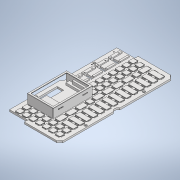
# Autodesk Inventor part: Backboard
Saved by Autodesk Inventor 2021 (Build 250183000, 183)
## iProperties
Created: 2020-06-05
Part Number: Backboard
Material: Generic
Document SubType Name: Modeling
Designer: ameli
Density: 1 g/cm^3
Appearance: Default
Author: ameli
Autodesk Inventor part; units mm, degrees
(part 1 of 4)
ref_plane "YZ Plane" through (0, 0, 0) normal (1, 0, 0) x (0, 1, 0)
ref_plane "XZ Plane" through (0, 0, 0) normal (0, 1, 0) x (-1, 0, 0)
sketch "Sketch1" plane through (0, 0, 0) normal (0, 1, 0) x (-1, 0, 0)
  line L0 (60.5, 128.25) -> (-60.5, 128.25)
  line L1 (-60.5, 128.25) -> (-60.5, -128.25)
  line L2 (-60.5, -128.25) -> (60.5, -128.25)
  line L3 (60.5, -128.25) -> (60.5, 128.25)
  point P0 (0, 0)
  dimension "d0" = 121
  dimension "d1" = 256.5
  dimension "d2" = 60.5
  dimension "d3" = 128.25
  constraints: 8 end point, 2 parallel, 1 horizontal, 1 perpendicular
  measures "d0" distance of L0.start L0.end
  measures "d1" distance of L2.end L0.start
  measures "d2" distance from line of point (0, 0) L3
  measures "d3" distance from line of point (0, 0) L0
extrude "Extrusion1" add sketch "Sketch1" along normal blind 4
sketch "Sketch10" plane through (0, 4, 0) normal (0, 1, 0) x (1, 0, 0)
  line L0 (-49.5, -119.5) -> (-41, -119.5)
  line L1 (-41, -119.5) -> (-41, -118)
  line L2 (-41, -118) -> (-49.5, -118)
  line L3 (-49.5, -118) -> (-49.5, -119.5)
  line L4 (-49.5, -107) -> (-41, -107)
  line L5 (-41, -107) -> (-41, -105.5)
  line L6 (-41, -105.5) -> (-49.5, -105.5)
  line L7 (-49.5, -105.5) -> (-49.5, -107)
  line L8 (-60.5, 128.25) -> (-60.5, -128.25) projected
  line L9 (-60.5, -128.25) -> (60.5, -128.25) projected
  line L10 (-49.5, -104.5) -> (-41, -104.5)
  line L11 (-41, -104.5) -> (-41, -103)
  line L12 (-41, -103) -> (-49.5, -103)
  line L13 (-49.5, -103) -> (-49.5, -104.5)
  line L14 (-49.5, -92) -> (-41, -92)
  line L15 (-41, -92) -> (-41, -90.5)
  line L16 (-41, -90.5) -> (-49.5, -90.5)
  line L17 (-49.5, -90.5) -> (-49.5, -92)
  line L18 (-49.5, -89.5) -> (-41, -89.5)
  line L19 (-41, -89.5) -> (-41, -88)
  line L20 (-41, -88) -> (-49.5, -88)
  line L21 (-49.5, -88) -> (-49.5, -89.5)
  line L22 (-49.5, -77) -> (-41, -77)
  line L23 (-41, -77) -> (-41, -75.5)
  line L24 (-41, -75.5) -> (-49.5, -75.5)
  line L25 (-49.5, -75.5) -> (-49.5, -77)
  line L26 (-49.5, -74.5) -> (-41, -74.5)
  line L27 (-41, -74.5) -> (-41, -73)
  line L28 (-41, -73) -> (-49.5, -73)
  line L29 (-49.5, -73) -> (-49.5, -74.5)
  line L30 (-49.5, -62) -> (-41, -62)
  line L31 (-41, -62) -> (-41, -60.5)
  line L32 (-41, -60.5) -> (-49.5, -60.5)
  line L33 (-49.5, -60.5) -> (-49.5, -62)
  line L34 (-49.5, -59.5) -> (-41, -59.5)
  line L35 (-41, -59.5) -> (-41, -58)
  line L36 (-41, -58) -> (-49.5, -58)
  line L37 (-49.5, -58) -> (-49.5, -59.5)
  line L38 (-49.5, -47) -> (-41, -47)
  line L39 (-41, -47) -> (-41, -45.5)
  line L40 (-41, -45.5) -> (-49.5, -45.5)
  line L41 (-49.5, -45.5) -> (-49.5, -47)
  line L42 (-49.5, -44.5) -> (-41, -44.5)
  line L43 (-41, -44.5) -> (-41, -43)
  line L44 (-41, -43) -> (-49.5, -43)
  line L45 (-49.5, -43) -> (-49.5, -44.5)
  line L46 (-49.5, -32) -> (-41, -32)
  line L47 (-41, -32) -> (-41, -30.5)
  line L48 (-41, -30.5) -> (-49.5, -30.5)
  line L49 (-49.5, -30.5) -> (-49.5, -32)
  line L50 (-49.5, -29.5) -> (-41, -29.5)
  line L51 (-41, -29.5) -> (-41, -28)
  line L52 (-41, -28) -> (-49.5, -28)
  line L53 (-49.5, -28) -> (-49.5, -29.5)
  line L54 (-49.5, -17) -> (-41, -17)
  line L55 (-41, -17) -> (-41, -15.5)
  line L56 (-41, -15.5) -> (-49.5, -15.5)
  line L57 (-49.5, -15.5) -> (-49.5, -17)
  line L58 (-49.5, -14.5) -> (-41, -14.5)
  line L59 (-41, -14.5) -> (-41, -13)
  line L60 (-41, -13) -> (-49.5, -13)
  line L61 (-49.5, -13) -> (-49.5, -14.5)
  line L62 (-49.5, -2) -> (-41, -2)
  line L63 (-41, -2) -> (-41, -0.5)
  line L64 (-41, -0.5) -> (-49.5, -0.5)
  line L65 (-49.5, -0.5) -> (-49.5, -2)
  line L66 (-49.5, 0.5) -> (-41, 0.5)
  line L67 (-41, 0.5) -> (-41, 2)
  line L68 (-41, 2) -> (-49.5, 2)
  line L69 (-49.5, 2) -> (-49.5, 0.5)
  line L70 (-49.5, 13) -> (-41, 13)
  line L71 (-41, 13) -> (-41, 14.5)
  line L72 (-41, 14.5) -> (-49.5, 14.5)
  line L73 (-49.5, 14.5) -> (-49.5, 13)
  line L74 (-49.5, 15.5) -> (-41, 15.5)
  line L75 (-41, 15.5) -> (-41, 17)
  line L76 (-41, 17) -> (-49.5, 17)
  line L77 (-49.5, 17) -> (-49.5, 15.5)
  line L78 (-49.5, 28) -> (-41, 28)
  line L79 (-41, 28) -> (-41, 29.5)
  line L80 (-41, 29.5) -> (-49.5, 29.5)
  line L81 (-49.5, 29.5) -> (-49.5, 28)
  line L82 (-49.5, 30.5) -> (-41, 30.5)
  line L83 (-41, 30.5) -> (-41, 32)
  line L84 (-41, 32) -> (-49.5, 32)
  line L85 (-49.5, 32) -> (-49.5, 30.5)
  line L86 (-49.5, 43) -> (-41, 43)
  line L87 (-41, 43) -> (-41, 44.5)
  line L88 (-41, 44.5) -> (-49.5, 44.5)
  line L89 (-49.5, 44.5) -> (-49.5, 43)
  line L90 (-49.5, 45.5) -> (-41, 45.5)
  line L91 (-41, 45.5) -> (-41, 47)
  line L92 (-41, 47) -> (-49.5, 47)
  line L93 (-49.5, 47) -> (-49.5, 45.5)
  line L94 (-49.5, 58) -> (-41, 58)
  line L95 (-41, 58) -> (-41, 59.5)
  line L96 (-41, 59.5) -> (-49.5, 59.5)
  line L97 (-49.5, 59.5) -> (-49.5, 58)
  line L98 (-49.5, 60.5) -> (-41, 60.5)
  line L99 (-41, 60.5) -> (-41, 62)
  line L100 (-41, 62) -> (-49.5, 62)
  line L101 (-49.5, 62) -> (-49.5, 60.5)
  line L102 (-49.5, 73) -> (-41, 73)
  line L103 (-41, 73) -> (-41, 74.5)
  line L104 (-41, 74.5) -> (-49.5, 74.5)
  line L105 (-49.5, 74.5) -> (-49.5, 73)
  line L106 (-49.5, 75.5) -> (-41, 75.5)
  line L107 (-41, 75.5) -> (-41, 77)
  line L108 (-41, 77) -> (-49.5, 77)
  line L109 (-49.5, 77) -> (-49.5, 75.5)
  line L110 (-49.5, 88) -> (-41, 88)
  line L111 (-41, 88) -> (-41, 89.5)
  line L112 (-41, 89.5) -> (-49.5, 89.5)
  line L113 (-49.5, 89.5) -> (-49.5, 88)
  line L114 (-49.5, 90.5) -> (-41, 90.5)
  line L115 (-41, 90.5) -> (-41, 92)
  line L116 (-41, 92) -> (-49.5, 92)
  line L117 (-49.5, 92) -> (-49.5, 90.5)
  line L118 (-49.5, 103) -> (-41, 103)
  line L119 (-41, 103) -> (-41, 104.5)
  line L120 (-41, 104.5) -> (-49.5, 104.5)
  line L121 (-49.5, 104.5) -> (-49.5, 103)
  line L122 (-49.5, 105.5) -> (-41, 105.5)
  line L123 (-41, 105.5) -> (-41, 107)
  line L124 (-41, 107) -> (-49.5, 107)
  line L125 (-49.5, 107) -> (-49.5, 105.5)
  line L126 (-49.5, 118) -> (-41, 118)
  line L127 (-41, 118) -> (-41, 119.5)
  line L128 (-41, 119.5) -> (-49.5, 119.5)
  line L129 (-49.5, 119.5) -> (-49.5, 118)
  line L130 (-34.5, -119.5) -> (-26, -119.5)
  line L131 (-26, -119.5) -> (-26, -118)
  line L132 (-26, -118) -> (-34.5, -118)
  line L133 (-34.5, -118) -> (-34.5, -119.5)
  line L134 (-34.5, -107) -> (-26, -107)
  line L135 (-26, -107) -> (-26, -105.5)
  line L136 (-26, -105.5) -> (-34.5, -105.5)
  line L137 (-34.5, -105.5) -> (-34.5, -107)
  line L138 (-34.5, -104.5) -> (-26, -104.5)
  line L139 (-26, -104.5) -> (-26, -103)
  line L140 (-26, -103) -> (-34.5, -103)
  line L141 (-34.5, -103) -> (-34.5, -104.5)
  line L142 (-34.5, -92) -> (-26, -92)
  line L143 (-26, -92) -> (-26, -90.5)
  line L144 (-26, -90.5) -> (-34.5, -90.5)
  line L145 (-34.5, -90.5) -> (-34.5, -92)
  line L146 (-34.5, -89.5) -> (-26, -89.5)
  line L147 (-26, -89.5) -> (-26, -88)
  line L148 (-26, -88) -> (-34.5, -88)
  line L149 (-34.5, -88) -> (-34.5, -89.5)
  line L150 (-34.5, -77) -> (-26, -77)
  line L151 (-26, -77) -> (-26, -75.5)
  line L152 (-26, -75.5) -> (-34.5, -75.5)
  line L153 (-34.5, -75.5) -> (-34.5, -77)
  line L154 (-34.5, -74.5) -> (-26, -74.5)
  line L155 (-26, -74.5) -> (-26, -73)
  line L156 (-26, -73) -> (-34.5, -73)
  line L157 (-34.5, -73) -> (-34.5, -74.5)
  line L158 (-34.5, -62) -> (-26, -62)
  line L159 (-26, -62) -> (-26, -60.5)
  line L160 (-26, -60.5) -> (-34.5, -60.5)
  line L161 (-34.5, -60.5) -> (-34.5, -62)
  line L162 (-34.5, -59.5) -> (-26, -59.5)
  line L163 (-26, -59.5) -> (-26, -58)
  line L164 (-26, -58) -> (-34.5, -58)
  line L165 (-34.5, -58) -> (-34.5, -59.5)
  line L166 (-34.5, -47) -> (-26, -47)
  line L167 (-26, -47) -> (-26, -45.5)
  line L168 (-26, -45.5) -> (-34.5, -45.5)
  line L169 (-34.5, -45.5) -> (-34.5, -47)
  line L170 (-34.5, -44.5) -> (-26, -44.5)
  line L171 (-26, -44.5) -> (-26, -43)
  line L172 (-26, -43) -> (-34.5, -43)
  line L173 (-34.5, -43) -> (-34.5, -44.5)
  line L174 (-34.5, -32) -> (-26, -32)
  line L175 (-26, -32) -> (-26, -30.5)
  line L176 (-26, -30.5) -> (-34.5, -30.5)
  line L177 (-34.5, -30.5) -> (-34.5, -32)
  line L178 (-34.5, -29.5) -> (-26, -29.5)
  line L179 (-26, -29.5) -> (-26, -28)
  line L180 (-26, -28) -> (-34.5, -28)
  line L181 (-34.5, -28) -> (-34.5, -29.5)
  line L182 (-34.5, -17) -> (-26, -17)
  line L183 (-26, -17) -> (-26, -15.5)
  line L184 (-26, -15.5) -> (-34.5, -15.5)
  line L185 (-34.5, -15.5) -> (-34.5, -17)
  line L186 (-34.5, -14.5) -> (-26, -14.5)
  line L187 (-26, -14.5) -> (-26, -13)
  line L188 (-26, -13) -> (-34.5, -13)
  line L189 (-34.5, -13) -> (-34.5, -14.5)
  line L190 (-34.5, -2) -> (-26, -2)
  line L191 (-26, -2) -> (-26, -0.5)
  line L192 (-26, -0.5) -> (-34.5, -0.5)
  line L193 (-34.5, -0.5) -> (-34.5, -2)
  line L194 (-34.5, 0.5) -> (-26, 0.5)
  line L195 (-26, 0.5) -> (-26, 2)
  line L196 (-26, 2) -> (-34.5, 2)
  line L197 (-34.5, 2) -> (-34.5, 0.5)
  line L198 (-34.5, 13) -> (-26, 13)
  line L199 (-26, 13) -> (-26, 14.5)
  line L200 (-26, 14.5) -> (-34.5, 14.5)
  line L201 (-34.5, 14.5) -> (-34.5, 13)
  line L202 (-34.5, 15.5) -> (-26, 15.5)
  line L203 (-26, 15.5) -> (-26, 17)
  line L204 (-26, 17) -> (-34.5, 17)
  line L205 (-34.5, 17) -> (-34.5, 15.5)
  line L206 (-34.5, 28) -> (-26, 28)
  line L207 (-26, 28) -> (-26, 29.5)
  line L208 (-26, 29.5) -> (-34.5, 29.5)
  line L209 (-34.5, 29.5) -> (-34.5, 28)
  line L210 (-34.5, 30.5) -> (-26, 30.5)
  line L211 (-26, 30.5) -> (-26, 32)
  line L212 (-26, 32) -> (-34.5, 32)
  line L213 (-34.5, 32) -> (-34.5, 30.5)
  line L214 (-34.5, 43) -> (-26, 43)
  line L215 (-26, 43) -> (-26, 44.5)
  line L216 (-26, 44.5) -> (-34.5, 44.5)
  line L217 (-34.5, 44.5) -> (-34.5, 43)
  line L218 (-34.5, 45.5) -> (-26, 45.5)
  line L219 (-26, 45.5) -> (-26, 47)
  line L220 (-26, 47) -> (-34.5, 47)
  line L221 (-34.5, 47) -> (-34.5, 45.5)
  line L222 (-34.5, 58) -> (-26, 58)
  line L223 (-26, 58) -> (-26, 59.5)
  line L224 (-26, 59.5) -> (-34.5, 59.5)
  line L225 (-34.5, 59.5) -> (-34.5, 58)
  line L226 (-34.5, 60.5) -> (-26, 60.5)
  line L227 (-26, 60.5) -> (-26, 62)
  line L228 (-26, 62) -> (-34.5, 62)
  line L229 (-34.5, 62) -> (-34.5, 60.5)
  line L230 (-34.5, 73) -> (-26, 73)
  line L231 (-26, 73) -> (-26, 74.5)
  line L232 (-26, 74.5) -> (-34.5, 74.5)
  line L233 (-34.5, 74.5) -> (-34.5, 73)
  line L234 (-34.5, 75.5) -> (-26, 75.5)
  line L235 (-26, 75.5) -> (-26, 77)
  line L236 (-26, 77) -> (-34.5, 77)
  line L237 (-34.5, 77) -> (-34.5, 75.5)
  line L238 (-34.5, 88) -> (-26, 88)
  line L239 (-26, 88) -> (-26, 89.5)
  line L240 (-26, 89.5) -> (-34.5, 89.5)
  line L241 (-34.5, 89.5) -> (-34.5, 88)
  line L242 (-34.5, 90.5) -> (-26, 90.5)
  line L243 (-26, 90.5) -> (-26, 92)
  line L244 (-26, 92) -> (-34.5, 92)
  line L245 (-34.5, 92) -> (-34.5, 90.5)
  line L246 (-34.5, 103) -> (-26, 103)
  line L247 (-26, 103) -> (-26, 104.5)
  line L248 (-26, 104.5) -> (-34.5, 104.5)
  line L249 (-34.5, 104.5) -> (-34.5, 103)
  line L250 (-34.5, 105.5) -> (-26, 105.5)
  line L251 (-26, 105.5) -> (-26, 107)
  line L252 (-26, 107) -> (-34.5, 107)
  line L253 (-34.5, 107) -> (-34.5, 105.5)
  line L254 (-34.5, 118) -> (-26, 118)
  line L255 (-26, 118) -> (-26, 119.5)
  line L256 (-26, 119.5) -> (-34.5, 119.5)
  line L257 (-34.5, 119.5) -> (-34.5, 118)
  line L258 (-19.5, -119.5) -> (-11, -119.5)
  line L259 (-11, -119.5) -> (-11, -118)
  line L260 (-11, -118) -> (-19.5, -118)
  line L261 (-19.5, -118) -> (-19.5, -119.5)
  line L262 (-19.5, -107) -> (-11, -107)
  line L263 (-11, -107) -> (-11, -105.5)
  line L264 (-11, -105.5) -> (-19.5, -105.5)
  line L265 (-19.5, -105.5) -> (-19.5, -107)
  line L266 (-19.5, -104.5) -> (-11, -104.5)
  line L267 (-11, -104.5) -> (-11, -103)
  line L268 (-11, -103) -> (-19.5, -103)
  line L269 (-19.5, -103) -> (-19.5, -104.5)
  line L270 (-19.5, -92) -> (-11, -92)
  line L271 (-11, -92) -> (-11, -90.5)
  line L272 (-11, -90.5) -> (-19.5, -90.5)
  line L273 (-19.5, -90.5) -> (-19.5, -92)
  line L274 (-19.5, -89.5) -> (-11, -89.5)
  line L275 (-11, -89.5) -> (-11, -88)
  line L276 (-11, -88) -> (-19.5, -88)
  line L277 (-19.5, -88) -> (-19.5, -89.5)
  line L278 (-19.5, -77) -> (-11, -77)
  line L279 (-11, -77) -> (-11, -75.5)
  line L280 (-11, -75.5) -> (-19.5, -75.5)
  line L281 (-19.5, -75.5) -> (-19.5, -77)
  line L282 (-19.5, -74.5) -> (-11, -74.5)
  line L283 (-11, -74.5) -> (-11, -73)
  line L284 (-11, -73) -> (-19.5, -73)
  line L285 (-19.5, -73) -> (-19.5, -74.5)
  line L286 (-19.5, -62) -> (-11, -62)
  line L287 (-11, -62) -> (-11, -60.5)
  line L288 (-11, -60.5) -> (-19.5, -60.5)
  line L289 (-19.5, -60.5) -> (-19.5, -62)
  line L290 (-19.5, -59.5) -> (-11, -59.5)
  line L291 (-11, -59.5) -> (-11, -58)
  line L292 (-11, -58) -> (-19.5, -58)
  line L293 (-19.5, -58) -> (-19.5, -59.5)
  line L294 (-19.5, -47) -> (-11, -47)
  line L295 (-11, -47) -> (-11, -45.5)
  line L296 (-11, -45.5) -> (-19.5, -45.5)
  line L297 (-19.5, -45.5) -> (-19.5, -47)
  line L298 (-19.5, -44.5) -> (-11, -44.5)
  line L299 (-11, -44.5) -> (-11, -43)
  line L300 (-11, -43) -> (-19.5, -43)
  line L301 (-19.5, -43) -> (-19.5, -44.5)
  line L302 (-19.5, -32) -> (-11, -32)
  line L303 (-11, -32) -> (-11, -30.5)
  line L304 (-11, -30.5) -> (-19.5, -30.5)
  line L305 (-19.5, -30.5) -> (-19.5, -32)
  line L306 (-19.5, -29.5) -> (-11, -29.5)
  line L307 (-11, -29.5) -> (-11, -28)
  line L308 (-11, -28) -> (-19.5, -28)
  line L309 (-19.5, -28) -> (-19.5, -29.5)
  line L310 (-19.5, -17) -> (-11, -17)
  line L311 (-11, -17) -> (-11, -15.5)
  line L312 (-11, -15.5) -> (-19.5, -15.5)
  line L313 (-19.5, -15.5) -> (-19.5, -17)
  line L314 (-19.5, -14.5) -> (-11, -14.5)
  line L315 (-11, -14.5) -> (-11, -13)
  line L316 (-11, -13) -> (-19.5, -13)
  line L317 (-19.5, -13) -> (-19.5, -14.5)
  line L318 (-19.5, -2) -> (-11, -2)
  line L319 (-11, -2) -> (-11, -0.5)
  line L320 (-11, -0.5) -> (-19.5, -0.5)
  line L321 (-19.5, -0.5) -> (-19.5, -2)
  line L322 (-19.5, 0.5) -> (-11, 0.5)
  line L323 (-11, 0.5) -> (-11, 2)
  line L324 (-11, 2) -> (-19.5, 2)
  line L325 (-19.5, 2) -> (-19.5, 0.5)
  line L326 (-19.5, 13) -> (-11, 13)
  line L327 (-11, 13) -> (-11, 14.5)
  line L328 (-11, 14.5) -> (-19.5, 14.5)
  line L329 (-19.5, 14.5) -> (-19.5, 13)
  line L330 (-19.5, 15.5) -> (-11, 15.5)
  line L331 (-11, 15.5) -> (-11, 17)
  line L332 (-11, 17) -> (-19.5, 17)
  line L333 (-19.5, 17) -> (-19.5, 15.5)
  line L334 (-19.5, 28) -> (-11, 28)
  line L335 (-11, 28) -> (-11, 29.5)
  line L336 (-11, 29.5) -> (-19.5, 29.5)
  line L337 (-19.5, 29.5) -> (-19.5, 28)
  line L338 (-19.5, 30.5) -> (-11, 30.5)
  line L339 (-11, 30.5) -> (-11, 32)
  line L340 (-11, 32) -> (-19.5, 32)
  line L341 (-19.5, 32) -> (-19.5, 30.5)
  line L342 (-19.5, 43) -> (-11, 43)
  line L343 (-11, 43) -> (-11, 44.5)
  line L344 (-11, 44.5) -> (-19.5, 44.5)
  line L345 (-19.5, 44.5) -> (-19.5, 43)
  line L346 (-19.5, 45.5) -> (-11, 45.5)
  line L347 (-11, 45.5) -> (-11, 47)
  line L348 (-11, 47) -> (-19.5, 47)
  line L349 (-19.5, 47) -> (-19.5, 45.5)
  line L350 (-19.5, 58) -> (-11, 58)
  line L351 (-11, 58) -> (-11, 59.5)
  line L352 (-11, 59.5) -> (-19.5, 59.5)
  line L353 (-19.5, 59.5) -> (-19.5, 58)
  line L354 (-19.5, 60.5) -> (-11, 60.5)
  line L355 (-11, 60.5) -> (-11, 62)
  line L356 (-11, 62) -> (-19.5, 62)
  line L357 (-19.5, 62) -> (-19.5, 60.5)
  line L358 (-19.5, 73) -> (-11, 73)
  line L359 (-11, 73) -> (-11, 74.5)
  line L360 (-11, 74.5) -> (-19.5, 74.5)
  line L361 (-19.5, 74.5) -> (-19.5, 73)
  line L362 (-19.5, 75.5) -> (-11, 75.5)
  line L363 (-11, 75.5) -> (-11, 77)
  line L364 (-11, 77) -> (-19.5, 77)
  line L365 (-19.5, 77) -> (-19.5, 75.5)
  line L366 (-19.5, 88) -> (-11, 88)
  line L367 (-11, 88) -> (-11, 89.5)
  line L368 (-11, 89.5) -> (-19.5, 89.5)
  line L369 (-19.5, 89.5) -> (-19.5, 88)
  line L370 (-19.5, 90.5) -> (-11, 90.5)
  line L371 (-11, 90.5) -> (-11, 92)
  line L372 (-11, 92) -> (-19.5, 92)
  line L373 (-19.5, 92) -> (-19.5, 90.5)
  line L374 (-19.5, 103) -> (-11, 103)
  line L375 (-11, 103) -> (-11, 104.5)
  line L376 (-11, 104.5) -> (-19.5, 104.5)
  line L377 (-19.5, 104.5) -> (-19.5, 103)
  line L378 (-19.5, 105.5) -> (-11, 105.5)
  line L379 (-11, 105.5) -> (-11, 107)
  line L380 (-11, 107) -> (-19.5, 107)
  line L381 (-19.5, 107) -> (-19.5, 105.5)
  line L382 (-19.5, 118) -> (-11, 118)
  line L383 (-11, 118) -> (-11, 119.5)
  line L384 (-11, 119.5) -> (-19.5, 119.5)
  line L385 (-19.5, 119.5) -> (-19.5, 118)
  line L386 (-4.5, -119.5) -> (4, -119.5)
  line L387 (4, -119.5) -> (4, -118)
  line L388 (4, -118) -> (-4.5, -118)
  line L389 (-4.5, -118) -> (-4.5, -119.5)
  line L390 (-4.5, -107) -> (4, -107)
  line L391 (4, -107) -> (4, -105.5)
  line L392 (4, -105.5) -> (-4.5, -105.5)
  line L393 (-4.5, -105.5) -> (-4.5, -107)
  line L394 (-4.5, -104.5) -> (4, -104.5)
  line L395 (4, -104.5) -> (4, -103)
  line L396 (4, -103) -> (-4.5, -103)
  line L397 (-4.5, -103) -> (-4.5, -104.5)
  line L398 (-4.5, -92) -> (4, -92)
  line L399 (4, -92) -> (4, -90.5)
  line L400 (4, -90.5) -> (-4.5, -90.5)
  line L401 (-4.5, -90.5) -> (-4.5, -92)
  line L402 (-4.5, -89.5) -> (4, -89.5)
  line L403 (4, -89.5) -> (4, -88)
  line L404 (4, -88) -> (-4.5, -88)
  line L405 (-4.5, -88) -> (-4.5, -89.5)
  line L406 (-4.5, -77) -> (4, -77)
  line L407 (4, -77) -> (4, -75.5)
  line L408 (4, -75.5) -> (-4.5, -75.5)
  line L409 (-4.5, -75.5) -> (-4.5, -77)
  line L410 (-4.5, -74.5) -> (4, -74.5)
  line L411 (4, -74.5) -> (4, -73)
  line L412 (4, -73) -> (-4.5, -73)
  line L413 (-4.5, -73) -> (-4.5, -74.5)
  line L414 (-4.5, -62) -> (4, -62)
  line L415 (4, -62) -> (4, -60.5)
  line L416 (4, -60.5) -> (-4.5, -60.5)
  line L417 (-4.5, -60.5) -> (-4.5, -62)
  line L418 (-4.5, -59.5) -> (4, -59.5)
  line L419 (4, -59.5) -> (4, -58)
  line L420 (4, -58) -> (-4.5, -58)
  line L421 (-4.5, -58) -> (-4.5, -59.5)
  line L422 (-4.5, -47) -> (4, -47)
  line L423 (4, -47) -> (4, -45.5)
  line L424 (4, -45.5) -> (-4.5, -45.5)
  line L425 (-4.5, -45.5) -> (-4.5, -47)
  line L426 (-4.5, -44.5) -> (4, -44.5)
  line L427 (4, -44.5) -> (4, -43)
  line L428 (4, -43) -> (-4.5, -43)
  line L429 (-4.5, -43) -> (-4.5, -44.5)
  line L430 (-4.5, -32) -> (4, -32)
  line L431 (4, -32) -> (4, -30.5)
  line L432 (4, -30.5) -> (-4.5, -30.5)
  line L433 (-4.5, -30.5) -> (-4.5, -32)
  line L434 (-4.5, -29.5) -> (4, -29.5)
  line L435 (4, -29.5) -> (4, -28)
  line L436 (4, -28) -> (-4.5, -28)
  line L437 (-4.5, -28) -> (-4.5, -29.5)
  line L438 (-4.5, -17) -> (4, -17)
  line L439 (4, -17) -> (4, -15.5)
  line L440 (4, -15.5) -> (-4.5, -15.5)
  line L441 (-4.5, -15.5) -> (-4.5, -17)
  line L442 (-4.5, -14.5) -> (4, -14.5)
  line L443 (4, -14.5) -> (4, -13)
  line L444 (4, -13) -> (-4.5, -13)
  line L445 (-4.5, -13) -> (-4.5, -14.5)
  line L446 (-4.5, -2) -> (4, -2)
  line L447 (4, -2) -> (4, -0.5)
  line L448 (4, -0.5) -> (-4.5, -0.5)
  line L449 (-4.5, -0.5) -> (-4.5, -2)
  line L450 (-4.5, 0.5) -> (4, 0.5)
  line L451 (4, 0.5) -> (4, 2)
  line L452 (4, 2) -> (-4.5, 2)
  line L453 (-4.5, 2) -> (-4.5, 0.5)
  line L454 (-4.5, 13) -> (4, 13)
  line L455 (4, 13) -> (4, 14.5)
  line L456 (4, 14.5) -> (-4.5, 14.5)
  line L457 (-4.5, 14.5) -> (-4.5, 13)
  line L458 (-4.5, 15.5) -> (4, 15.5)
  line L459 (4, 15.5) -> (4, 17)
  line L460 (4, 17) -> (-4.5, 17)
  line L461 (-4.5, 17) -> (-4.5, 15.5)
  line L462 (-4.5, 28) -> (4, 28)
  line L463 (4, 28) -> (4, 29.5)
  line L464 (4, 29.5) -> (-4.5, 29.5)
  line L465 (-4.5, 29.5) -> (-4.5, 28)
  line L466 (-4.5, 30.5) -> (4, 30.5)
  line L467 (4, 30.5) -> (4, 32)
  line L468 (4, 32) -> (-4.5, 32)
  line L469 (-4.5, 32) -> (-4.5, 30.5)
  line L470 (-4.5, 43) -> (4, 43)
  line L471 (4, 43) -> (4, 44.5)
  line L472 (4, 44.5) -> (-4.5, 44.5)
  line L473 (-4.5, 44.5) -> (-4.5, 43)
  line L474 (-4.5, 45.5) -> (4, 45.5)
  line L475 (4, 45.5) -> (4, 47)
  line L476 (4, 47) -> (-4.5, 47)
  line L477 (-4.5, 47) -> (-4.5, 45.5)
  line L478 (-4.5, 58) -> (4, 58)
  line L479 (4, 58) -> (4, 59.5)
  line L480 (4, 59.5) -> (-4.5, 59.5)
  line L481 (-4.5, 59.5) -> (-4.5, 58)
  line L482 (-4.5, 60.5) -> (4, 60.5)
  line L483 (4, 60.5) -> (4, 62)
  line L484 (4, 62) -> (-4.5, 62)
  line L485 (-4.5, 62) -> (-4.5, 60.5)
  line L486 (-4.5, 73) -> (4, 73)
  line L487 (4, 73) -> (4, 74.5)
  line L488 (4, 74.5) -> (-4.5, 74.5)
  line L489 (-4.5, 74.5) -> (-4.5, 73)
  line L490 (-4.5, 75.5) -> (4, 75.5)
  line L491 (4, 75.5) -> (4, 77)
  line L492 (4, 77) -> (-4.5, 77)
  line L493 (-4.5, 77) -> (-4.5, 75.5)
  line L494 (-4.5, 88) -> (4, 88)
  line L495 (4, 88) -> (4, 89.5)
  line L496 (4, 89.5) -> (-4.5, 89.5)
  line L497 (-4.5, 89.5) -> (-4.5, 88)
  line L498 (-4.5, 90.5) -> (4, 90.5)
  line L499 (4, 90.5) -> (4, 92)
  line L500 (4, 92) -> (-4.5, 92)
  line L501 (-4.5, 92) -> (-4.5, 90.5)
  line L502 (-4.5, 103) -> (4, 103)
  line L503 (4, 103) -> (4, 104.5)
  line L504 (4, 104.5) -> (-4.5, 104.5)
  line L505 (-4.5, 104.5) -> (-4.5, 103)
  line L506 (-4.5, 105.5) -> (4, 105.5)
  line L507 (4, 105.5) -> (4, 107)
  line L508 (4, 107) -> (-4.5, 107)
  line L509 (-4.5, 107) -> (-4.5, 105.5)
  line L510 (-4.5, 118) -> (4, 118)
  line L511 (4, 118) -> (4, 119.5)
  line L512 (4, 119.5) -> (-4.5, 119.5)
  line L513 (-4.5, 119.5) -> (-4.5, 118)
  line L514 (10.5, -119.5) -> (19, -119.5)
  line L515 (19, -119.5) -> (19, -118)
  line L516 (19, -118) -> (10.5, -118)
  line L517 (10.5, -118) -> (10.5, -119.5)
  line L518 (10.5, -107) -> (19, -107)
  line L519 (19, -107) -> (19, -105.5)
  line L520 (19, -105.5) -> (10.5, -105.5)
  line L521 (10.5, -105.5) -> (10.5, -107)
  line L522 (10.5, -104.5) -> (19, -104.5)
  line L523 (19, -104.5) -> (19, -103)
  line L524 (19, -103) -> (10.5, -103)
  line L525 (10.5, -103) -> (10.5, -104.5)
  line L526 (10.5, -92) -> (19, -92)
  line L527 (19, -92) -> (19, -90.5)
  line L528 (19, -90.5) -> (10.5, -90.5)
  line L529 (10.5, -90.5) -> (10.5, -92)
  line L530 (10.5, -89.5) -> (19, -89.5)
  line L531 (19, -89.5) -> (19, -88)
  line L532 (19, -88) -> (10.5, -88)
  line L533 (10.5, -88) -> (10.5, -89.5)
  line L534 (10.5, -77) -> (19, -77)
  line L535 (19, -77) -> (19, -75.5)
  line L536 (19, -75.5) -> (10.5, -75.5)
  line L537 (10.5, -75.5) -> (10.5, -77)
  line L538 (10.5, -74.5) -> (19, -74.5)
  line L539 (19, -74.5) -> (19, -73)
  line L540 (19, -73) -> (10.5, -73)
  line L541 (10.5, -73) -> (10.5, -74.5)
  line L542 (10.5, -62) -> (19, -62)
  line L543 (19, -62) -> (19, -60.5)
  line L544 (19, -60.5) -> (10.5, -60.5)
  line L545 (10.5, -60.5) -> (10.5, -62)
  line L546 (10.5, -59.5) -> (19, -59.5)
  line L547 (19, -59.5) -> (19, -58)
  line L548 (19, -58) -> (10.5, -58)
  line L549 (10.5, -58) -> (10.5, -59.5)
  line L550 (10.5, -47) -> (19, -47)
  line L551 (19, -47) -> (19, -45.5)
  line L552 (19, -45.5) -> (10.5, -45.5)
  line L553 (10.5, -45.5) -> (10.5, -47)
  line L554 (10.5, -44.5) -> (19, -44.5)
  line L555 (19, -44.5) -> (19, -43)
  line L556 (19, -43) -> (10.5, -43)
  line L557 (10.5, -43) -> (10.5, -44.5)
  line L558 (10.5, -32) -> (19, -32)
  line L559 (19, -32) -> (19, -30.5)
  line L560 (19, -30.5) -> (10.5, -30.5)
  line L561 (10.5, -30.5) -> (10.5, -32)
  line L562 (10.5, -29.5) -> (19, -29.5)
  line L563 (19, -29.5) -> (19, -28)
  line L564 (19, -28) -> (10.5, -28)
  line L565 (10.5, -28) -> (10.5, -29.5)
  line L566 (10.5, -17) -> (19, -17)
  line L567 (19, -17) -> (19, -15.5)
  line L568 (19, -15.5) -> (10.5, -15.5)
  line L569 (10.5, -15.5) -> (10.5, -17)
  line L570 (10.5, -14.5) -> (19, -14.5)
  line L571 (19, -14.5) -> (19, -13)
  line L572 (19, -13) -> (10.5, -13)
  line L573 (10.5, -13) -> (10.5, -14.5)
  line L574 (10.5, -2) -> (19, -2)
  line L575 (19, -2) -> (19, -0.5)
  line L576 (19, -0.5) -> (10.5, -0.5)
  line L577 (10.5, -0.5) -> (10.5, -2)
  line L578 (10.5, 0.5) -> (19, 0.5)
  line L579 (19, 0.5) -> (19, 2)
  line L580 (19, 2) -> (10.5, 2)
  line L581 (10.5, 2) -> (10.5, 0.5)
  line L582 (10.5, 13) -> (19, 13)
  line L583 (19, 13) -> (19, 14.5)
  line L584 (19, 14.5) -> (10.5, 14.5)
  line L585 (10.5, 14.5) -> (10.5, 13)
  line L586 (10.5, 15.5) -> (19, 15.5)
  line L587 (19, 15.5) -> (19, 17)
  line L588 (19, 17) -> (10.5, 17)
  line L589 (10.5, 17) -> (10.5, 15.5)
  line L590 (10.5, 28) -> (19, 28)
  line L591 (19, 28) -> (19, 29.5)
  line L592 (19, 29.5) -> (10.5, 29.5)
  line L593 (10.5, 29.5) -> (10.5, 28)
  line L594 (10.5, 30.5) -> (19, 30.5)
  line L595 (19, 30.5) -> (19, 32)
  line L596 (19, 32) -> (10.5, 32)
  line L597 (10.5, 32) -> (10.5, 30.5)
  line L598 (10.5, 43) -> (19, 43)
  line L599 (19, 43) -> (19, 44.5)
  line L600 (19, 44.5) -> (10.5, 44.5)
  line L601 (10.5, 44.5) -> (10.5, 43)
  line L602 (10.5, 45.5) -> (19, 45.5)
  line L603 (19, 45.5) -> (19, 47)
  line L604 (19, 47) -> (10.5, 47)
  line L605 (10.5, 47) -> (10.5, 45.5)
  line L606 (10.5, 58) -> (19, 58)
  line L607 (19, 58) -> (19, 59.5)
  line L608 (19, 59.5) -> (10.5, 59.5)
  line L609 (10.5, 59.5) -> (10.5, 58)
  line L610 (10.5, 60.5) -> (19, 60.5)
  line L611 (19, 60.5) -> (19, 62)
  line L612 (19, 62) -> (10.5, 62)
  line L613 (10.5, 62) -> (10.5, 60.5)
  line L614 (10.5, 73) -> (19, 73)
  line L615 (19, 73) -> (19, 74.5)
  line L616 (19, 74.5) -> (10.5, 74.5)
  line L617 (10.5, 74.5) -> (10.5, 73)
  line L618 (10.5, 75.5) -> (19, 75.5)
  line L619 (19, 75.5) -> (19, 77)
  line L620 (19, 77) -> (10.5, 77)
  line L621 (10.5, 77) -> (10.5, 75.5)
  line L622 (10.5, 88) -> (19, 88)
  line L623 (19, 88) -> (19, 89.5)
  line L624 (19, 89.5) -> (10.5, 89.5)
  line L625 (10.5, 89.5) -> (10.5, 88)
  line L626 (10.5, 90.5) -> (19, 90.5)
  line L627 (19, 90.5) -> (19, 92)
  line L628 (19, 92) -> (10.5, 92)
  line L629 (10.5, 92) -> (10.5, 90.5)
  line L630 (10.5, 103) -> (19, 103)
  line L631 (19, 103) -> (19, 104.5)
  line L632 (19, 104.5) -> (10.5, 104.5)
  line L633 (10.5, 104.5) -> (10.5, 103)
  line L634 (10.5, 105.5) -> (19, 105.5)
  line L635 (19, 105.5) -> (19, 107)
  line L636 (19, 107) -> (10.5, 107)
  line L637 (10.5, 107) -> (10.5, 105.5)
  line L638 (10.5, 118) -> (19, 118)
  line L639 (19, 118) -> (19, 119.5)
  line L640 (19, 119.5) -> (10.5, 119.5)
  line L641 (10.5, 119.5) -> (10.5, 118)
  line L642 (25.5, -119.5) -> (34, -119.5)
  line L643 (34, -119.5) -> (34, -118)
  line L644 (34, -118) -> (25.5, -118)
  line L645 (25.5, -118) -> (25.5, -119.5)
  line L646 (25.5, -107) -> (34, -107)
  line L647 (34, -107) -> (34, -105.5)
  line L648 (34, -105.5) -> (25.5, -105.5)
  line L649 (25.5, -105.5) -> (25.5, -107)
  line L650 (25.5, -104.5) -> (34, -104.5)
  line L651 (34, -104.5) -> (34, -103)
  line L652 (34, -103) -> (25.5, -103)
  line L653 (25.5, -103) -> (25.5, -104.5)
  line L654 (25.5, -92) -> (34, -92)
  line L655 (34, -92) -> (34, -90.5)
  line L656 (34, -90.5) -> (25.5, -90.5)
  line L657 (25.5, -90.5) -> (25.5, -92)
  line L658 (25.5, -89.5) -> (34, -89.5)
  line L659 (34, -89.5) -> (34, -88)
  line L660 (34, -88) -> (25.5, -88)
  line L661 (25.5, -88) -> (25.5, -89.5)
  line L662 (25.5, -77) -> (34, -77)
  line L663 (34, -77) -> (34, -75.5)
  line L664 (34, -75.5) -> (25.5, -75.5)
  line L665 (25.5, -75.5) -> (25.5, -77)
  line L666 (25.5, -74.5) -> (34, -74.5)
  line L667 (34, -74.5) -> (34, -73)
  line L668 (34, -73) -> (25.5, -73)
  line L669 (25.5, -73) -> (25.5, -74.5)
  line L670 (25.5, -62) -> (34, -62)
  line L671 (34, -62) -> (34, -60.5)
  line L672 (34, -60.5) -> (25.5, -60.5)
  line L673 (25.5, -60.5) -> (25.5, -62)
  line L674 (25.5, -59.5) -> (34, -59.5)
  line L675 (34, -59.5) -> (34, -58)
  line L676 (34, -58) -> (25.5, -58)
  line L677 (25.5, -58) -> (25.5, -59.5)
  line L678 (25.5, -47) -> (34, -47)
  line L679 (34, -47) -> (34, -45.5)
  line L680 (34, -45.5) -> (25.5, -45.5)
  line L681 (25.5, -45.5) -> (25.5, -47)
  line L682 (25.5, -44.5) -> (34, -44.5)
  line L683 (34, -44.5) -> (34, -43)
  line L684 (34, -43) -> (25.5, -43)
  line L685 (25.5, -43) -> (25.5, -44.5)
  line L686 (25.5, -32) -> (34, -32)
  line L687 (34, -32) -> (34, -30.5)
  line L688 (34, -30.5) -> (25.5, -30.5)
  line L689 (25.5, -30.5) -> (25.5, -32)
  line L690 (25.5, -29.5) -> (34, -29.5)
  line L691 (34, -29.5) -> (34, -28)
  line L692 (34, -28) -> (25.5, -28)
  line L693 (25.5, -28) -> (25.5, -29.5)
  line L694 (25.5, -17) -> (34, -17)
  line L695 (34, -17) -> (34, -15.5)
  line L696 (34, -15.5) -> (25.5, -15.5)
  line L697 (25.5, -15.5) -> (25.5, -17)
  line L698 (25.5, -14.5) -> (34, -14.5)
  line L699 (34, -14.5) -> (34, -13)
  line L700 (34, -13) -> (25.5, -13)
  line L701 (25.5, -13) -> (25.5, -14.5)
  line L702 (25.5, -2) -> (34, -2)
  line L703 (34, -2) -> (34, -0.5)
  line L704 (34, -0.5) -> (25.5, -0.5)
  line L705 (25.5, -0.5) -> (25.5, -2)
  line L706 (25.5, 0.5) -> (34, 0.5)
  line L707 (34, 0.5) -> (34, 2)
  line L708 (34, 2) -> (25.5, 2)
  line L709 (25.5, 2) -> (25.5, 0.5)
  line L710 (25.5, 13) -> (34, 13)
  line L711 (34, 13) -> (34, 14.5)
  line L712 (34, 14.5) -> (25.5, 14.5)
  line L713 (25.5, 14.5) -> (25.5, 13)
  line L714 (25.5, 15.5) -> (34, 15.5)
  line L715 (34, 15.5) -> (34, 17)
  line L716 (34, 17) -> (25.5, 17)
  line L717 (25.5, 17) -> (25.5, 15.5)
  line L718 (25.5, 28) -> (34, 28)
  line L719 (34, 28) -> (34, 29.5)
  line L720 (34, 29.5) -> (25.5, 29.5)
  line L721 (25.5, 29.5) -> (25.5, 28)
  line L722 (25.5, 30.5) -> (34, 30.5)
  line L723 (34, 30.5) -> (34, 32)
  line L724 (34, 32) -> (25.5, 32)
  line L725 (25.5, 32) -> (25.5, 30.5)
  line L726 (25.5, 43) -> (34, 43)
  line L727 (34, 43) -> (34, 44.5)
  line L728 (34, 44.5) -> (25.5, 44.5)
  line L729 (25.5, 44.5) -> (25.5, 43)
  line L730 (25.5, 45.5) -> (34, 45.5)
  line L731 (34, 45.5) -> (34, 47)
  line L732 (34, 47) -> (25.5, 47)
  line L733 (25.5, 47) -> (25.5, 45.5)
  line L734 (25.5, 58) -> (34, 58)
  line L735 (34, 58) -> (34, 59.5)
  line L736 (34, 59.5) -> (25.5, 59.5)
  line L737 (25.5, 59.5) -> (25.5, 58)
  line L738 (25.5, 60.5) -> (34, 60.5)
  line L739 (34, 60.5) -> (34, 62)
  line L740 (34, 62) -> (25.5, 62)
  line L741 (25.5, 62) -> (25.5, 60.5)
  line L742 (25.5, 73) -> (34, 73)
  line L743 (34, 73) -> (34, 74.5)
  line L744 (34, 74.5) -> (25.5, 74.5)
  line L745 (25.5, 74.5) -> (25.5, 73)
  line L746 (25.5, 75.5) -> (34, 75.5)
  line L747 (34, 75.5) -> (34, 77)
  line L748 (34, 77) -> (25.5, 77)
  line L749 (25.5, 77) -> (25.5, 75.5)
  line L750 (25.5, 88) -> (34, 88)
  line L751 (34, 88) -> (34, 89.5)
  line L752 (34, 89.5) -> (25.5, 89.5)
  line L753 (25.5, 89.5) -> (25.5, 88)
  line L754 (25.5, 90.5) -> (34, 90.5)
  line L755 (34, 90.5) -> (34, 92)
  line L756 (34, 92) -> (25.5, 92)
  line L757 (25.5, 92) -> (25.5, 90.5)
  line L758 (25.5, 103) -> (34, 103)
  line L759 (34, 103) -> (34, 104.5)
  line L760 (34, 104.5) -> (25.5, 104.5)
  line L761 (25.5, 104.5) -> (25.5, 103)
  line L762 (25.5, 105.5) -> (34, 105.5)
  line L763 (34, 105.5) -> (34, 107)
  line L764 (34, 107) -> (25.5, 107)
  line L765 (25.5, 107) -> (25.5, 105.5)
  line L766 (25.5, 118) -> (34, 118)
  line L767 (34, 118) -> (34, 119.5)
  line L768 (34, 119.5) -> (25.5, 119.5)
  line L769 (25.5, 119.5) -> (25.5, 118)
  line L770 (40.5, -119.5) -> (49, -119.5)
  line L771 (49, -119.5) -> (49, -118)
  line L772 (49, -118) -> (40.5, -118)
  line L773 (40.5, -118) -> (40.5, -119.5)
  line L774 (40.5, -107) -> (49, -107)
  line L775 (49, -107) -> (49, -105.5)
  line L776 (49, -105.5) -> (40.5, -105.5)
  line L777 (40.5, -105.5) -> (40.5, -107)
  line L778 (40.5, -104.5) -> (49, -104.5)
  line L779 (49, -104.5) -> (49, -103)
  line L780 (49, -103) -> (40.5, -103)
  line L781 (40.5, -103) -> (40.5, -104.5)
  line L782 (40.5, -92) -> (49, -92)
  line L783 (49, -92) -> (49, -90.5)
  line L784 (49, -90.5) -> (40.5, -90.5)
  line L785 (40.5, -90.5) -> (40.5, -92)
  line L786 (40.5, -89.5) -> (49, -89.5)
  line L787 (49, -89.5) -> (49, -88)
  line L788 (49, -88) -> (40.5, -88)
  line L789 (40.5, -88) -> (40.5, -89.5)
  line L790 (40.5, -77) -> (49, -77)
  line L791 (49, -77) -> (49, -75.5)
  line L792 (49, -75.5) -> (40.5, -75.5)
  line L793 (40.5, -75.5) -> (40.5, -77)
  line L794 (40.5, -74.5) -> (49, -74.5)
  line L795 (49, -74.5) -> (49, -73)
  line L796 (49, -73) -> (40.5, -73)
  line L797 (40.5, -73) -> (40.5, -74.5)
  line L798 (40.5, -62) -> (49, -62)
  line L799 (49, -62) -> (49, -60.5)
  line L800 (49, -60.5) -> (40.5, -60.5)
  line L801 (40.5, -60.5) -> (40.5, -62)
  line L802 (40.5, -59.5) -> (49, -59.5)
  line L803 (49, -59.5) -> (49, -58)
  line L804 (49, -58) -> (40.5, -58)
  line L805 (40.5, -58) -> (40.5, -59.5)
  line L806 (40.5, -47) -> (49, -47)
  line L807 (49, -47) -> (49, -45.5)
  line L808 (49, -45.5) -> (40.5, -45.5)
  line L809 (40.5, -45.5) -> (40.5, -47)
  line L810 (40.5, -44.5) -> (49, -44.5)
  line L811 (49, -44.5) -> (49, -43)
  line L812 (49, -43) -> (40.5, -43)
  line L813 (40.5, -43) -> (40.5, -44.5)
  line L814 (40.5, -32) -> (49, -32)
  line L815 (49, -32) -> (49, -30.5)
  line L816 (49, -30.5) -> (40.5, -30.5)
  line L817 (40.5, -30.5) -> (40.5, -32)
  line L818 (40.5, -29.5) -> (49, -29.5)
  line L819 (49, -29.5) -> (49, -28)
  line L820 (49, -28) -> (40.5, -28)
  line L821 (40.5, -28) -> (40.5, -29.5)
  line L822 (40.5, -17) -> (49, -17)
  line L823 (49, -17) -> (49, -15.5)
  line L824 (49, -15.5) -> (40.5, -15.5)
  line L825 (40.5, -15.5) -> (40.5, -17)
  line L826 (40.5, -14.5) -> (49, -14.5)
  line L827 (49, -14.5) -> (49, -13)
  line L828 (49, -13) -> (40.5, -13)
  line L829 (40.5, -13) -> (40.5, -14.5)
  line L830 (40.5, -2) -> (49, -2)
  line L831 (49, -2) -> (49, -0.5)
  line L832 (49, -0.5) -> (40.5, -0.5)
  line L833 (40.5, -0.5) -> (40.5, -2)
  line L834 (40.5, 0.5) -> (49, 0.5)
  line L835 (49, 0.5) -> (49, 2)
  line L836 (49, 2) -> (40.5, 2)
  line L837 (40.5, 2) -> (40.5, 0.5)
  line L838 (40.5, 13) -> (49, 13)
  line L839 (49, 13) -> (49, 14.5)
  line L840 (49, 14.5) -> (40.5, 14.5)
  line L841 (40.5, 14.5) -> (40.5, 13)
  line L842 (40.5, 15.5) -> (49, 15.5)
  line L843 (49, 15.5) -> (49, 17)
  line L844 (49, 17) -> (40.5, 17)
  line L845 (40.5, 17) -> (40.5, 15.5)
  line L846 (40.5, 28) -> (49, 28)
  line L847 (49, 28) -> (49, 29.5)
  line L848 (49, 29.5) -> (40.5, 29.5)
  line L849 (40.5, 29.5) -> (40.5, 28)
  line L850 (40.5, 30.5) -> (49, 30.5)
  line L851 (49, 30.5) -> (49, 32)
  line L852 (49, 32) -> (40.5, 32)
  line L853 (40.5, 32) -> (40.5, 30.5)
  line L854 (40.5, 43) -> (49, 43)
  line L855 (49, 43) -> (49, 44.5)
  line L856 (49, 44.5) -> (40.5, 44.5)
  line L857 (40.5, 44.5) -> (40.5, 43)
  line L858 (40.5, 45.5) -> (49, 45.5)
  line L859 (49, 45.5) -> (49, 47)
  line L860 (49, 47) -> (40.5, 47)
  line L861 (40.5, 47) -> (40.5, 45.5)
  line L862 (40.5, 58) -> (49, 58)
  line L863 (49, 58) -> (49, 59.5)
  line L864 (49, 59.5) -> (40.5, 59.5)
  line L865 (40.5, 59.5) -> (40.5, 58)
  line L866 (40.5, 60.5) -> (49, 60.5)
  line L867 (49, 60.5) -> (49, 62)
  line L868 (49, 62) -> (40.5, 62)
  line L869 (40.5, 62) -> (40.5, 60.5)
  line L870 (40.5, 73) -> (49, 73)
  line L871 (49, 73) -> (49, 74.5)
  line L872 (49, 74.5) -> (40.5, 74.5)
  line L873 (40.5, 74.5) -> (40.5, 73)
  line L874 (40.5, 75.5) -> (49, 75.5)
  line L875 (49, 75.5) -> (49, 77)
  line L876 (49, 77) -> (40.5, 77)
  line L877 (40.5, 77) -> (40.5, 75.5)
  line L878 (40.5, 88) -> (49, 88)
  line L879 (49, 88) -> (49, 89.5)
  line L880 (49, 89.5) -> (40.5, 89.5)
  line L881 (40.5, 89.5) -> (40.5, 88)
  line L882 (40.5, 90.5) -> (49, 90.5)
  line L883 (49, 90.5) -> (49, 92)
  line L884 (49, 92) -> (40.5, 92)
  line L885 (40.5, 92) -> (40.5, 90.5)
  line L886 (40.5, 103) -> (49, 103)
  line L887 (49, 103) -> (49, 104.5)
  line L888 (49, 104.5) -> (40.5, 104.5)
  line L889 (40.5, 104.5) -> (40.5, 103)
  line L890 (40.5, 105.5) -> (49, 105.5)
  line L891 (49, 105.5) -> (49, 107)
  line L892 (49, 107) -> (40.5, 107)
  line L893 (40.5, 107) -> (40.5, 105.5)
  line L894 (40.5, 118) -> (49, 118)
  line L895 (49, 118) -> (49, 119.5)
  line L896 (49, 119.5) -> (40.5, 119.5)
  line L897 (40.5, 119.5) -> (40.5, 118)
  line L898 (60.5, -128.25) -> (60.5, 128.25) projected
  line L899 (10.5, -69.5) -> (19, -69.5)
  line L900 (19, -69.5) -> (19, -68)
  line L901 (19, -68) -> (10.5, -68)
  line L902 (10.5, -68) -> (10.5, -69.5)
  line L903 (10.5, -67) -> (19, -67)
  line L904 (19, -67) -> (19, -65.5)
  line L905 (19, -65.5) -> (10.5, -65.5)
  line L906 (10.5, -65.5) -> (10.5, -67)
  line L907 (10.5, -24.5) -> (19, -24.5)
  line L908 (19, -24.5) -> (19, -23)
  line L909 (19, -23) -> (10.5, -23)
  line L910 (10.5, -23) -> (10.5, -24.5)
  line L911 (10.5, -22) -> (19, -22)
  line L912 (19, -22) -> (19, -20.5)
  line L913 (19, -20.5) -> (10.5, -20.5)
  line L914 (10.5, -20.5) -> (10.5, -22)
  line L915 (10.5, -9.5) -> (19, -9.5)
  line L916 (19, -9.5) -> (19, -8)
  line L917 (19, -8) -> (10.5, -8)
  line L918 (10.5, -8) -> (10.5, -9.5)
  line L919 (10.5, -7) -> (19, -7)
  line L920 (19, -7) -> (19, -5.5)
  line L921 (19, -5.5) -> (10.5, -5.5)
  line L922 (10.5, -5.5) -> (10.5, -7)
  line L923 (10.5, 35.5) -> (19, 35.5)
  line L924 (19, 35.5) -> (19, 37)
  line L925 (19, 37) -> (10.5, 37)
  line L926 (10.5, 37) -> (10.5, 35.5)
  line L927 (10.5, 38) -> (19, 38)
  line L928 (19, 38) -> (19, 39.5)
  line L929 (19, 39.5) -> (10.5, 39.5)
  line L930 (10.5, 39.5) -> (10.5, 38)
  line L931 (10.5, 80.5) -> (19, 80.5)
  line L932 (19, 80.5) -> (19, 82)
  line L933 (19, 82) -> (10.5, 82)
  line L934 (10.5, 82) -> (10.5, 80.5)
  line L935 (10.5, 83) -> (19, 83)
  line L936 (19, 83) -> (19, 84.5)
  line L937 (19, 84.5) -> (10.5, 84.5)
  line L938 (10.5, 84.5) -> (10.5, 83)
  line L939 (10.5, 95.5) -> (19, 95.5)
  line L940 (19, 95.5) -> (19, 97)
  line L941 (19, 97) -> (10.5, 97)
  line L942 (10.5, 97) -> (10.5, 95.5)
  line L943 (10.5, 98) -> (19, 98)
  line L944 (19, 98) -> (19, 99.5)
  line L945 (19, 99.5) -> (10.5, 99.5)
  line L946 (10.5, 99.5) -> (10.5, 98)
  point P0 (0, 0)
  dimension "d93" = 8.5
  dimension "d94" = 1.5
  dimension "d95" = 1.5
  dimension "d96" = 11
  dimension "d97" = 11
  dimension "d98" = 8.75
  dimension "d101" = 15
  dimension "d104" = 15
  dimension "d249" = 18.5
  dimension "d250" = 1.5
  dimension "d251" = 8.5
  dimension "d252" = 1.5
  dimension "d253" = 18.5
  dimension "d254" = 1.5
  dimension "d255" = 1.5
  dimension "d256" = 1.5
  dimension "d257" = 8.5
  dimension "d258" = 18.5
  dimension "d259" = 8.5
  dimension "d260" = 11
  dimension "d261" = 1
  dimension "d262" = 8.5
  dimension "d263" = 18.5
  dimension "d264" = 1.5
  dimension "d265" = 1.5
  dimension "d266" = 1.5
  dimension "d267" = 18.5
  dimension "d268" = 18.5
  dimension "d269" = 8.5
  dimension "d270" = 8.5
  dimension "d271" = 1.5
  dimension "d272" = 1.5
  dimension "d273" = 1.5
  dimension "d274" = 1.5
  dimension "d275" = 18.5
  dimension "d276" = 1
  dimension "d277" = 18.5
  dimension "d278" = 1
  dimension "d279" = 8.5
  dimension "d280" = 8.5
  dimension "d281" = 8.5
  dimension "d282" = 8.5
  constraints: 1888 end point, 238 point on line, 28 parallel, 15 horizontal, 14 perpendicular, 1 vertical, 1776 other
  measures "d93" distance of L5.end L6.end
  measures "d94" distance of L2.end L0.start
  measures "d95" distance of L6.end L4.start
  measures "d96" distance between parallel lines of L2 L4
  measures "d97" distance between parallel lines of L8 L3
  measures "d98" distance between parallel lines of L9 L0
  measures "d101" distance of L0.start L10.start
  measures "d104" distance of L0.start L130.start
  measures "d249" distance between parallel lines of L899 L532
  measures "d250" distance of L901.end L899.start
  measures "d251" distance between parallel lines of L539 L902
  measures "d252" distance of L905.end L903.start
  measures "d253" distance between parallel lines of L550 L905
  measures "d254" distance of L909.end L907.start
  measures "d255" distance of L913.end L911.start
  measures "d256" distance of L917.end L915.start
  measures "d257" distance between parallel lines of L545 L904
  measures "d258" distance between parallel lines of L556 L907
  measures "d259" distance between parallel lines of L563 L910
  measures "d260" distance between parallel lines of L915 L913
  measures "d261" distance between parallel lines of L909 L911
  measures "d262" distance between parallel lines of L565 L908
  measures "d263" distance between parallel lines of L582 L921
  measures "d264" distance of L919.end L920.end
  measures "d265" distance of L925.end L923.start
  measures "d266" distance of L929.end L927.start
  measures "d267" distance between parallel lines of L588 L923
  measures "d268" distance between parallel lines of L606 L929
  measures "d269" distance between parallel lines of L601 L928
  measures "d270" distance between parallel lines of L599 L930
  measures "d271" distance of L933.end L931.start
  measures "d272" distance of L937.end L935.start
  measures "d273" distance of L941.end L939.start
  measures "d274" distance of L945.end L943.start
  measures "d275" distance between parallel lines of L638 L945
  measures "d276" distance between parallel lines of L941 L943
  measures "d277" distance between parallel lines of L612 L931
  measures "d278" distance between parallel lines of L933 L935
  measures "d279" distance between parallel lines of L619 L934
  measures "d280" distance between parallel lines of L625 L932
  measures "d281" distance between parallel lines of L627 L942
  measures "d282" distance between parallel lines of L633 L944
extrude "Extrusion4" cut sketch "Sketch10" against normal through all contours L3 L2 L1 L0 | L7 L6 L5 L4 | L13 L12 L11 L10 | L17 L16 L15 L14 | L133 L132 L131 L130 | L137 L136 L135 L134 | L141 L140 L139 L138 | L145 L144 L143 L142 | L261 L260 L259 L258 | L265 L264 L263 L262 | L269 L268 L267 L266 | L273 L272 L271 L270 | L325 L324 L323 L322 | L329 L328 L327 L326 | L333 L332 L331 L330 | L337 L336 L335 L334 | L341 L340 L339 L338 | L345 L344 L343 L342 | L349 L348 L347 L346 | L353 L352 L351 L350 | L357 L356 L355 L354 | L361 L360 L359 L358 | L365 L364 L363 L362 | L369 L368 L367 L366 | L373 L372 L371 L370 | L377 L376 L375 L374 | L381 L380 L379 L378 | L385 L384 L383 L382 | L389 L388 L387 L386 | L393 L392 L391 L390 | L397 L396 L395 L394 | L401 L400 L399 L398 | L453 L452 L451 L450 | L457 L456 L455 L454 | L461 L460 L459 L458 | L465 L464 L463 L462 | L469 L468 L467 L466 | L473 L472 L471 L470 | L477 L476 L475 L474 | L481 L480 L479 L478 | L485 L484 L483 L482 | L489 L488 L487 L486 | L493 L492 L491 L490 | L497 L496 L495 L494 | L501 L500 L499 L498 | L505 L504 L503 L502 | L509 L508 L507 L506 | L513 L512 L511 L510 | L517 L516 L515 L514 | L521 L520 L519 L518 | L525 L524 L523 L522 | L529 L528 L527 L526 | L533 L532 L531 L530 | L553 L552 L551 L550 | L557 L556 L555 L554 | L585 L584 L583 L582 | L589 L588 L587 L586 | L609 L608 L607 L606 | L613 L612 L611 L610 | L641 L640 L639 L638 | L645 L644 L643 L642 | L649 L648 L647 L646 | L653 L652 L651 L650 | L657 L656 L655 L654 | L661 L660 L659 L658 | L665 L664 L663 L662 | L669 L668 L667 L666 | L673 L672 L671 L670 | L677 L676 L675 L674 | L681 L680 L679 L678 | L685 L684 L683 L682 | L689 L688 L687 L686 | L693 L692 L691 L690 | L697 L696 L695 L694 | L701 L700 L699 L698 | L705 L704 L703 L702 | L709 L708 L707 L706 | L713 L712 L711 L710 | L717 L716 L715 L714 | L721 L720 L719 L718 | L725 L724 L723 L722 | L729 L728 L727 L726 | L733 L732 L731 L730 | L737 L736 L735 L734 | L741 L740 L739 L738 | L745 L744 L743 L742 | L749 L748 L747 L746 | L753 L752 L751 L750 | L757 L756 L755 L754 | L761 L760 L759 L758 | L765 L764 L763 L762 | L769 L768 L767 L766 | L773 L772 L771 L770 | L777 L776 L775 L774 | L781 L780 L779 L778 | L785 L784 L783 L782 | L789 L788 L787 L786 | L793 L792 L791 L790 | L797 L796 L795 L794 | L801 L800 L799 L798 | L805 L804 L803 L802 | L809 L808 L807 L806 | L813 L812 L811 L810 | L817 L816 L815 L814 | L821 L820 L819 L818 | L825 L824 L823 L822 | L829 L828 L827 L826 | L833 L832 L831 L830 | L837 L836 L835 L834 | L841 L840 L839 L838 | L845 L844 L843 L842 | L849 L848 L847 L846 | L853 L852 L851 L850 | L857 L856 L855 L854 | L861 L860 L859 L858 | L865 L864 L863 L862 | L869 L868 L867 L866 | L873 L872 L871 L870 | L877 L876 L875 L874 | L881 L880 L879 L878 | L885 L884 L883 L882 | L889 L888 L887 L886 | L893 L892 L891 L890 | L897 L896 L895 L894 | L902 L901 L900 L899 | L906 L905 L904 L903 | L910 L909 L908 L907 | L914 L913 L912 L911 | L918 L917 L916 L915 | L922 L921 L920 L919 | L926 L925 L924 L923 | L930 L929 L928 L927 | L934 L933 L932 L931 | L938 L937 L936 L935 | L942 L941 L940 L939 | L946 L945 L944 L943